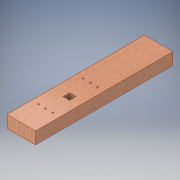
# Autodesk Inventor part: BO03
Saved by Autodesk Inventor 2017 (Build 210142000, 142)
## iProperties
Created: 2018-10-18
Part Number: BO03
Material: Wood (Oak)
Document SubType Name: Modeling
Designer: Dell
Density: 0.76 g/cm^3
Appearance: White Oak - Natural Medium Gloss
Author: Dell
Autodesk Inventor part; units mm, degrees
ref_plane "YZ Plane" through (0, 0, 0) normal (1, 0, 0) x (0, 1, 0)
ref_plane "XZ Plane" through (0, 0, 0) normal (0, 1, 0) x (-1, 0, 0)
ref_plane "XY Plane" through (0, 0, 0) normal (0, 0, 1) x (1, 0, 0)
sketch "Sketch1" plane through (0, 0, 0) normal (0, 0, 1) x (1, 0, 0)
  line L0 (0, 0) -> (88.9, 0)
  line L1 (88.9, 0) -> (88.9, 38.1)
  line L2 (88.9, 38.1) -> (0, 38.1)
  line L3 (0, 38.1) -> (0, 0)
  dimension "d0" = 88.9
  dimension "d1" = 38.1
  constraints: 8 end point, 2 parallel, 1 horizontal, 1 perpendicular
  measures "d0" distance of L2.end L1.end
  measures "d1" distance of L1.end L0.end
extrude "Extrusion1" add sketch "Sketch1" along normal blind 429.732
sketch "Sketch2" plane through (0, 38.1, 0) normal (0, 1, 0) x (1, 0, 0)
  line L0 (66.95, -353.532) -> (21.95, -353.532) construction
  line L1 (21.95, -353.532) -> (21.95, -213.532) construction
  line L2 (21.95, -213.532) -> (66.95, -213.532) construction
  line L3 (66.95, -213.532) -> (66.95, -353.532) construction
  circle A0 centre (21.95, -353.532) radius 2.3812
  circle A1 centre (44.45, -353.532) radius 2.3812
  circle A2 centre (66.95, -353.532) radius 2.3812
  circle A3 centre (66.95, -213.532) radius 2.3813
  circle A4 centre (44.45, -213.532) radius 2.3813
  circle A5 centre (21.95, -213.532) radius 2.3813
  line L4 (44.45, -353.532) -> (44.45, -213.532) construction
  line L5 (21.95, -283.532) -> (66.95, -283.532) construction
  line L6 (88.9, -429.732) -> (0, -429.732) projected
  line L7 (39.45, -293.532) -> (59.45, -293.532)
  line L8 (59.45, -293.532) -> (59.45, -273.532)
  line L9 (59.45, -273.532) -> (39.45, -273.532)
  line L10 (39.45, -273.532) -> (39.45, -293.532)
  point P0 (0, 0)
  point P1 (44.45, -429.732)
  dimension "d4" = 45
  dimension "d5" = 140
  dimension "d6" = 4.7625
  dimension "d7" = 4.7625
  dimension "d8" = 4.7625
  dimension "d9" = 4.7625
  dimension "d10" = 4.7625
  dimension "d11" = 4.7625
  dimension "d12" = 76.2
  dimension "d13" = 60
  dimension "d14" = 7.5
  dimension "d15" = 20
  dimension "d16" = 20
  constraints: 20 end point, 6 centre point, 5 midpoint, 4 coincident, 4 parallel, 2 horizontal, 2 perpendicular, 1 vertical, 1 vertical alignment
  measures "d4" distance of L1.end L2.end
  measures "d5" distance of L0.end L1.end
  measures "d6" diameter of A0
  measures "d7" diameter of A1
  measures "d8" diameter of A2
  measures "d9" diameter of A3
  measures "d10" diameter of A4
  measures "d11" diameter of A5
  measures "d12" distance between parallel lines of L6 L0
  measures "d13" distance from line of L4.end L9
  measures "d14" distance between parallel lines of L3 L8
  measures "d15" distance of L9.end L7.start
  measures "d16" distance of L7.start L7.end
extrude "Extrusion2" cut sketch "Sketch2" against normal through all
body "Solid1"
